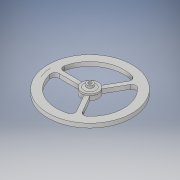
# Autodesk Inventor part: FlyWheel
Saved by Autodesk Inventor 2018 (Build 220112000, 112)
## iProperties
Created: 2019-06-12
Part Number: FlyWheel
Material: Generic
Document SubType Name: Modeling
Designer: anirudh
Density: 1 g/cm^3
Appearance: Default
Author: anirudh
Autodesk Inventor part; units mm, degrees
ref_plane "YZ Plane" through (0, 0, 0) normal (1, 0, 0) x (0, 1, 0)
ref_plane "XZ Plane" through (0, 0, 0) normal (0, 1, 0) x (-1, 0, 0)
ref_plane "XY Plane" through (0, 0, 0) normal (0, 0, 1) x (1, 0, 0)
sketch "Sketch1" plane through (0, 0, 0) normal (0, 1, 0) x (-1, 0, 0)
  circle A0 centre (0.043299, 0.009238) radius 63.5
  circle A1 centre (0.043299, 0.009238) radius 3.175
  line L0 (-31.236173, 47.839324) -> (-5.45384, 3.183013)
  line L1 (-25.739034, 51.013099) -> (0.041885, 6.359238)
  line L2 (57.105105, 3.183013) -> (5.543268, 3.183013)
  line L3 (57.105105, -3.164537) -> (5.540439, -3.164537)
  line L4 (-25.739034, -50.994622) -> (0.043299, -6.338311)
  line L5 (-31.236173, -47.820848) -> (-5.45384, -3.164537)
  arc A2 (5.543268, 3.183013) -> (0.041885, 6.359238) centre (0.043299, 0.009238) ccw
  arc A3 (-5.455254, 3.185463) -> (-5.455254, -3.166987) centre (0.043299, 0.009238) ccw
  arc A4 (0.041885, -6.340762) -> (5.543268, -3.164537) centre (0.043299, 0.009238) ccw
  arc A5 (57.105105, 3.183013) -> (-25.739034, 51.013099) centre (0.043299, 0.009238) ccw
  arc A6 (-31.236173, 47.839324) -> (-31.236173, -47.820848) centre (0.043299, 0.009238) ccw
  arc A7 (-25.739034, -50.994622) -> (57.105105, -3.164537) centre (0.043299, 0.009238) ccw
  constraints: 12 end point, 12 point on circle, 8 centre point, 4 point on line, 3 coincident, 2 horizontal
extrude "Extrusion2" add sketch "Sketch1" along normal blind 6.35
sketch "Sketch3" plane through (-0.043299, 6.35, 0.009238) normal (0, 1, 0) x (1, 0, 0)
  circle A0 centre (0.043299, 0.009238) radius 57.193746
  circle A1 centre (0.043299, 0.009238) radius 50.8
  point P0 (-57.061806, -3.173775)
  dimension "d25" = 101.6
  constraints: 2 coincident, 1 centre point, 3 other
  measures "d25" diameter of A1
extrude "Extrusion3" add sketch "Sketch3" against normal blind 6.35
fillet "Fillet3" radius 6.35 6 edges at (22.564, 3.175, 45.5138) (28.0638, 3.175, 42.3446) (-50.7002, 3.175, 3.183) (-50.7013, 3.175, -3.1645) (22.5723, 3.175, -45.5097) (28.0715, 3.175, -42.3395)
sketch "Sketch4" plane through (-0.043299, 6.35, 0.009238) normal (0, 1, 0) x (1, 0, 0)
  arc A0 (-5.499968, -3.173775) -> (0.001415, -6.35) centre (0, 0) ccw
  circle A1 centre (0, 0) radius 6.35
  circle A2 centre (0, 0) radius 9.525
  point P0 (-1.298596, -6.215798)
  point P1 (-4.733741, -4.232517)
  dimension "d29" = 19.05
  constraints: 2 centre point, 1 coincident, 1 point on circle
  measures "d29" diameter of A2
extrude "Extrusion4" add sketch "Sketch4" against normal blind 6.35
sketch "Sketch5" plane through (-0.043299, 6.35, 0.009238) normal (0, 1, 0) x (1, 0, 0)
  circle A0 centre (0, 0) radius 6.35
  dimension "d32" = 12.7
  constraints: 1 centre point
  measures "d32" diameter of A0
extrude "Extrusion5" cut sketch "Sketch5" against normal blind 6.35
sketch "Sketch6" plane through (-0.043299, 6.35, 0.009238) normal (0, 1, 0) x (1, 0, 0)
  circle A0 centre (0, 0) radius 6.35
  circle A1 centre (0, 0) radius 12.7
  dimension "d35" = 25.4
  constraints: 2 centre point, 1 coincident
  measures "d35" diameter of A1
extrude "Extrusion6" add sketch "Sketch6" against normal blind 6.35
ref_plane "Work Plane2" through (-0.043299, 8.8138, 0.009238) normal (0, 1, 0) x (1, 0, 0)
sketch "Sketch10" plane through (-0.043299, 8.8138, 0.009238) normal (0, 1, 0) x (1, 0, 0)
  circle A0 centre (0, 0) radius 6.35 projected
  circle A1 centre (0, 0) radius 2.54
  circle A2 centre (0, 0) radius 5.08
  dimension "d48" = 5.08
  dimension "d49" = 10.16
  constraints: 2 centre point, 2 coincident
  measures "d48" diameter of A1
  measures "d49" diameter of A2
extrude "Extrusion8" add sketch "Sketch10" along normal blind 5.3086 contours A2
sketch "Sketch12" plane through (0, 0, 0) normal (0, 0, 1) x (1, 0, 0)
  line L0 (-5.123299, 8.8138) -> (5.036701, 8.8138)
  line L1 (5.036701, 14.1224) -> (-5.123299, 14.1224)
  line L2 (63.456701, 6.35) -> (-63.543299, 6.35)
  line L3 (-0.043299, 6.35) -> (-6.393299, 6.35)
  line L4 (-6.393299, 6.35) -> (-6.393299, 8.1788)
  line L5 (-5.123299, 8.8138) -> (-5.123299, 14.1224)
  line L6 (-5.123299, 10.7188) -> (-5.123299, 8.8138)
  line L7 (-8.933299, 8.8138) -> (-12.743299, 8.8138)
  line L8 (-12.743299, 8.8138) -> (-12.743299, 6.35)
  line L9 (-12.743299, 6.35) -> (-6.393299, 6.35)
  line L10 (-0.043299, 16.94688) -> (-0.043299, -2.82448)
  line L11 (-8.933299, 8.8138) -> (-6.393299, 10.0838)
  line L12 (-5.123299, 8.8138) -> (-6.393299, 8.1788)
  line L13 (-8.933299, 8.8138) -> (-5.123299, 10.7188)
  line L14 (-12.743299, 8.8138) -> (-12.743299, 6.35)
  line L15 (-12.743299, 6.35) -> (-6.393299, 6.35)
  line L16 (-6.393299, 6.35) -> (-6.393299, 8.1788)
  line L17 (-6.393299, 8.1788) -> (-5.123299, 8.8138)
  line L18 (-5.123299, 8.8138) -> (-5.123299, 10.7188)
  line L19 (-5.123299, 10.7188) -> (-8.933299, 8.8138)
  line L20 (-8.933299, 8.8138) -> (-12.743299, 8.8138)
  point P0 (0, 0)
  dimension "d53" = 6.35
  constraints: 32 end point, 6 perpendicular, 2 parallel, 2 point on line, 1 collinear, 1 midpoint
  measures "d53" distance of L3.start L3.end
revolve "Revolution2" add sketch "Sketch12" angle 360 about axis through (-0.043299, 6.35, 0) along (0, -1, 0) contours L12 L4 L2 L8 L7 L11 L13 L5
sketch "Sketch13" plane through (-0.043299, 0, 0.009238) normal (0, -1, 0) x (1, 0, 0)
  circle A0 centre (0.043299, -0.009238) radius 5.715
  dimension "d64" = 11.43
  constraints: 1 centre point, 1 coincident
  measures "d64" diameter of A0
extrude "Extrusion9" cut sketch "Sketch13" against normal blind 8.8138
body "Solid2"
